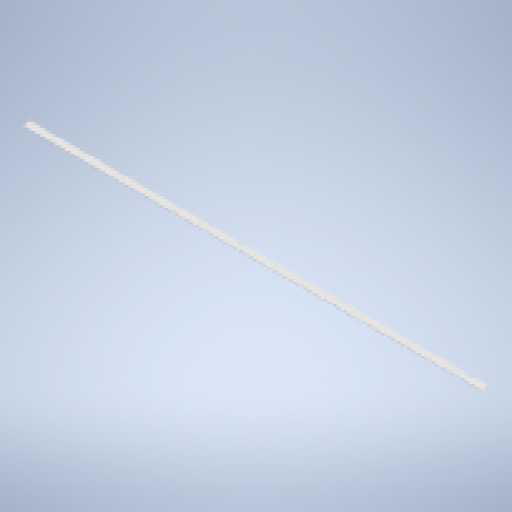
# Autodesk Inventor part: BSH 031 stringer floor
Saved by Autodesk Inventor 2025 (Build 290162010, 162A)
## iProperties
Created: 2024-07-23
Part Number: BSH 031 stringer floor
Material: 09g2s
Document SubType Name: Sheet Metal
Designer: pokla
Mass: 5330.4 g
Surface Area: 4696.25 cm^2
Volume: 679.031 cm^3
Density: 7.85 g/cm^3
Flat Pattern Width: 298 cm
Flat Pattern Length: 5 cm
Flat Pattern Area: 1490 cm^2
Sheet Metal Rule: AISI304 3mm Die 32
Sheet Metal Width: 2980,000 mm
Sheet Metal Length: 50,000 mm
Sheet Metal Area: 149000,000 mm^2
Appearance: Default
Stock Number: БШК 031 стрингер пол
Author: admin
Autodesk Inventor part; units mm, degrees
ref_plane "YZ Plane" through (0, 0, 0) normal (1, 0, 0) x (0, 1, 0)
ref_plane "XZ Plane" through (0, 0, 0) normal (0, 1, 0) x (-1, 0, 0)
ref_plane "XY Plane" through (0, 0, 0) normal (0, 0, 1) x (1, 0, 0)
sketch "Sketch8" plane through (0, 0, 0) normal (0, 0, 1) x (1, 0, 0)
  line L0 (-1490, 50) -> (1490, 50)
  line L1 (1490, 50) -> (1490, 0)
  line L2 (1490, 0) -> (-1490, 0)
  line L3 (-1490, 0) -> (-1490, 50)
  point P0 (0, 0)
  point P1 (0, 0)
  dimension "d37" = 50
  dimension "d38" = 2980
  measures "d37" distance of L2.end L0.start
  measures "d38" distance of L0.start L0.end
extrude "Plate5" add sketch "Sketch8" against normal blind 3
sketch "Sketch9" plane through (0, 0, 0) normal (0, 0, 1) x (1, 0, 0)
  line L0 (1490, 50) -> (-1490, 50) projected
  line L1 (-1374, 50) -> (-1370.8, 50)
  line L2 (-1370.8, 50) -> (-1370.8, 24)
  line L3 (-1370.8, 24) -> (-1374, 24)
  line L4 (-1374, 24) -> (-1374, 50)
  point P0 (0, 0)
  point P1 (-1370.8, 50)
  dimension "d40" = 116
  dimension "d41" = 3.2
  dimension "d42" = 26
  constraints: 8 end point, 2 parallel, 1 horizontal, 1 perpendicular, 1 point on line
  measures "d40" distance of L1.start L0.end
  measures "d41" distance between parallel lines of L4 L2
  measures "d42" distance of L1.end L2.end
extrude "Extrusion3" cut sketch "Sketch9" against normal through all
pattern_linear "Rectangular Pattern2" count 6 spacing 500 along (1, 0, 0) of "Extrusion3"
sketch "Sketch10" plane through (0, 0, -3) normal (0, 0, -1) x (-1, 0, 0)
  line L0 (-626, 50) -> (-626, 24) projected
  line L1 (-626, 24) -> (-629.2, 24) projected
  line L2 (-629.2, 24) -> (-629.2, 50) projected
  line L3 (-1490, 50) -> (-1129.2, 50) projected
  line L4 (-1490, 0) -> (-1490, 50) projected
  line L5 (1490, 0) -> (-1490, 0) projected
  line L6 (1490, 50) -> (1490, 0) projected
  line L7 (1374, 50) -> (1490, 50) projected
  line L8 (1374, 50) -> (1374, 24) projected
  line L9 (1374, 24) -> (1370.8, 24) projected
  line L10 (1370.8, 24) -> (1370.8, 50) projected
  line L11 (874, 50) -> (1370.8, 50) projected
  line L12 (874, 50) -> (874, 24) projected
  line L13 (874, 24) -> (870.8, 24) projected
  line L14 (870.8, 24) -> (870.8, 50) projected
  line L15 (374, 50) -> (870.8, 50) projected
  line L16 (374, 50) -> (374, 24) projected
  line L17 (374, 24) -> (370.8, 24) projected
  line L18 (370.8, 24) -> (370.8, 50) projected
  line L19 (-126, 50) -> (370.8, 50) projected
  line L20 (-126, 50) -> (-126, 24) projected
  line L21 (-126, 24) -> (-129.2, 24) projected
  line L22 (-129.2, 24) -> (-129.2, 50) projected
  line L23 (-626, 50) -> (-129.2, 50) projected
  circle A0 centre (115, 50) radius 20
  line L24 (374, 50) -> (870.8, 50) projected
  circle A1 centre (-1365, 50) radius 20
  line L25 (-1126, 50) -> (-1126, 24) projected
  line L26 (-1126, 24) -> (-1129.2, 24) projected
  line L27 (-1129.2, 24) -> (-1129.2, 50) projected
  line L28 (-1126, 50) -> (-629.2, 50) projected
  point P0 (0, 0)
  point P1 (770, 50)
  point P2 (730, 50)
  point P3 (-710, 50)
  point P4 (-750, 50)
  point P5 (-1345, 50)
  point P6 (-1385, 50)
  dimension "d48" = 40
  dimension "d49" = 40
  dimension "d50" = 1480
  dimension "d51" = 125
  constraints: 4 point on line, 2 centre point
  measures "d48" diameter of A0
  measures "d49" diameter of A1
  measures "d50" distance of A0.centre A1.centre
  measures "d51" distance from line of L4 A1.centre
extrude "Extrusion4" cut sketch "Sketch10" against normal through all contours A0 L19 | L19 A0 | A1 L3 | L3 A1
sketch "Sketch11" plane through (0, 0, -3) normal (0, 0, -1) x (-1, 0, 0)
  line L0 (-1348.785, 6.8732) -> (-1348.785, 21.8732) construction
  line L1 (-1348.785, 21.8732) -> (-1148.785, 21.8732) construction
  line L2 (-1148.785, 21.8732) -> (-1148.785, 6.8732) construction
  line L3 (-1148.785, 6.8732) -> (-1348.785, 6.8732) construction
  point P0 (0, 0)
  dimension "d54" = 200
  dimension "d55" = 15
  constraints: 1 horizontal, 2 other
  measures "d54" distance of L0.end L1.end
  measures "d55" distance between parallel lines of L1 L3
mark "Mark1"
equation "\"d39\" = Thickness"
equation "\"BendReliefWidth\" = Thickness"
equation "\"BendReliefDepth\" = 0.5 * Thickness"
equation "\"CornerReliefSize\" = 4 * Thickness"
equation "\"MinimumRemnant\" = 2 * Thickness"
equation "\"TransitionRadius\" = BendRadius"
equation "\"JacobiRadiusSize\" = BendRadius"
equation "\"GapSize\" = Thickness"
equation "\"Thickness\" = 3"
equation "\"BendRadius\" = 5"
body "Solid3"
